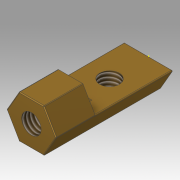
# Autodesk Inventor part: standoff
Saved by Autodesk Inventor 2019.3 (Build 233278000, 278)
## iProperties
Created: 2019-06-07
Part Number: standoff
Material: Generic
Document SubType Name: Modeling
Designer: Dave
Density: 1 g/cm^3
Appearance: Default
Author: Dave
Autodesk Inventor part; units mm, degrees
ref_plane "YZ Plane" through (0, 0, 0) normal (1, 0, 0) x (0, 1, 0)
ref_plane "XZ Plane" through (0, 0, 0) normal (0, 1, 0) x (-1, 0, 0)
ref_plane "XY Plane" through (0, 0, 0) normal (0, 0, 1) x (1, 0, 0)
sketch "Sketch1" plane through (0, 0, 0) normal (0, 0, 1) x (1, 0, 0)
  point P0 (0, 0)
sketch "Sketch2" plane through (0, 0, 0) normal (0, 0, 1) x (1, 0, 0)
  line L0 (3.1754, 0) -> (1.5877, -2.75)
  line L1 (1.5877, -2.75) -> (-1.5877, -2.75)
  line L2 (-1.5877, -2.75) -> (-3.1754, 0)
  line L3 (-3.1754, 0) -> (-1.5877, 2.75)
  line L4 (-1.5877, 2.75) -> (1.5877, 2.75)
  line L5 (1.5877, 2.75) -> (3.1754, 0)
  point P0 (0, 0)
  point P1 (0, 0)
  dimension "d0" = 5.5
  constraints: 12 end point, 1 coincident, 1 horizontal alignment, 13 other
  measures "d0" distance between parallel lines of L0 L3
extrude "Extrusion1" add sketch "Sketch2" along normal blind 15
sketch "Sketch3" plane through (0, 0, 15) normal (0, 0, 1) x (1, 0, 0)
  line L0 (1.5877, -2.75) -> (3.1754, 0) projected
  line L1 (3.1754, 0) -> (1.5877, 2.75) projected
  line L2 (1.5877, 2.75) -> (-1.5877, 2.75) projected
  line L3 (-1.5877, 2.75) -> (-3.1754, 0) projected
  line L4 (-3.1754, 0) -> (-1.5877, -2.75) projected
  line L5 (-1.5877, -2.75) -> (1.5877, -2.75) projected
  circle A0 centre (0, 0) radius 1.25
  dimension "d3" = 2.5
  constraints: 1 centre point, 1 coincident
  measures "d3" diameter of A0
extrude "Extrusion2" cut sketch "Sketch3" against normal blind 6.5 contours A0
thread "Thread1" size "M3x0.5" class "6H" standard "ANSI Metric M Profile" full length
sketch "Sketch4" plane through (0, 0, 0) normal (0, 1, 0) x (-1, 0, 0)
  line L0 (3.1754, 0) -> (3.1754, 15) projected
  line L1 (-3.1754, 0) -> (-3.1754, 15) projected
  line L2 (3.1754, 10) -> (-3.1754, 10)
  line L3 (-3.1754, 10) -> (-3.1754, 0)
  line L4 (-3.1754, 0) -> (3.1754, 0)
  line L5 (3.1754, 0) -> (3.1754, 10)
  line L6 (-1.5877, 15) -> (1.5877, 15) projected
  point P0 (0, 0)
  dimension "d8" = 5
  constraints: 8 end point, 2 parallel, 1 horizontal, 1 perpendicular, 1 point on line
  measures "d8" distance between parallel lines of L2 L6
extrude "Extrusion3" cut sketch "Sketch4" along normal blind 6.5
sketch "Sketch5" plane through (0, 0, 0) normal (0, 1, 0) x (1, 0, 0)
  circle A0 centre (0, -5) radius 1.25
  line L0 (1.5877, -15) -> (-1.5877, -15) projected
  line L1 (-3.1754, 0) -> (3.1754, 0) projected
  point P0 (0, 0)
  point P1 (0, 0)
  dimension "d11" = 2.5
  dimension "d12" = 10
  constraints: 1 centre point, 1 midpoint, 1 vertical alignment
  measures "d11" diameter of A0
  measures "d12" distance from line of L0 A0.centre
extrude "Extrusion4" cut sketch "Sketch5" against normal blind 6.5
thread "Thread2" size "M3x0.5" class "6H" standard "ANSI Metric M Profile" full length
fillet "Fillet1" radius 0.1 10 edges at (0, 0, 0) (2.3816, -1.375, 0) (0, -2.75, 0) (-2.3816, -1.375, 0) (2.3816, -1.375, 15) (2.3816, 1.375, 15) (0, 2.75, 15) (-2.3816, 1.375, 15) (-2.3816, -1.375, 15) (0, -2.75, 15)
fillet "Fillet2" radius 0.1 18 edges at (3.1416, 0, 14.9707) (3.1754, 0, 12.45) (3.1247, -0.0293, 0.0293) (3.1754, 0, 5.05) (1.5708, -2.7207, 14.9707) (1.5708, -2.7207, 0.0293) (1.5877, -2.75, 7.5) (-1.5708, -2.7207, 14.9707) (-1.5708, -2.7207, 0.0293) (-1.5877, -2.75, 7.5) (-3.1247, -0.0293, 0.0293) (-3.1754, 0, 5.05) (-3.1416, 0, 14.9707) (-3.1754, 0, 12.45) (-1.5708, 2.7207, 14.9707) (-1.5877, 2.75, 12.45) (1.5708, 2.7207, 14.9707) (1.5877, 2.75, 12.45)
body "Solid1"
